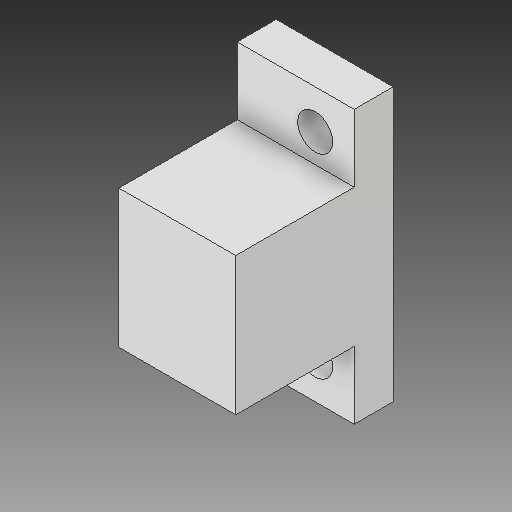
# Autodesk Inventor part: RailMount
Saved by Autodesk Inventor 2019.3 (Build 233278000, 278)
## iProperties
Created: 2019-06-25
Part Number: RailMount
Material: PC/ABS Plastic
Document SubType Name: Modeling
Designer: mark
Density: 0.357273 g/cm^3
Appearance: Smooth - White
Author: mark
Autodesk Inventor part; units mm, degrees
ref_plane "YZ Plane" through (0, 0, 0) normal (1, 0, 0) x (0, 1, 0)
ref_plane "XZ Plane" through (0, 0, 0) normal (0, 1, 0) x (-1, 0, 0)
ref_plane "XY Plane" through (0, 0, 0) normal (0, 0, 1) x (1, 0, 0)
sketch "Sketch1" plane through (0, 0, 0) normal (0, 0, 1) x (1, 0, 0)
  circle A0 centre (-50, 5.188) radius 4.5 projected
  circle A1 centre (-50, -44.812) radius 4.5 projected
  circle A2 centre (50, 5.188) radius 4.5 projected
  circle A3 centre (50, -44.812) radius 4.5 projected
  line L0 (30, 15.188) -> (60, 15.188)
  line L1 (60, 15.188) -> (60, -54.812)
  line L2 (60, -54.812) -> (30, -54.812)
  line L3 (30, -54.812) -> (30, 15.188)
  circle A4 centre (50, 5.188) radius 4
  circle A5 centre (50, -44.812) radius 4
  point P0 (0, 0)
  dimension "d1" = 30
  dimension "d2" = 60
  dimension "d28" = 10
  dimension "d29" = 10
  constraints: 8 end point, 2 centre point, 2 coincident, 2 horizontal, 2 vertical
  measures "d1" distance between parallel lines of L1 L3
  measures "d2" distance from line of point (0, 0) L1
  measures "d28" distance from line of L0 A2.centre
  measures "d29" distance from line of L2 A3.centre
extrude "Extrusion1" add sketch "Sketch1" along normal blind 10 contours L0 L1 L2 L3
sketch "Sketch2" plane through (0, 0, 10) normal (0, 0, 1) x (1, 0, 0)
  line L0 (60, -2.112) -> (55, -2.112)
  line L1 (55, -2.112) -> (55, -37.512)
  line L2 (55, -37.512) -> (60, -37.512)
  line L3 (60, -37.512) -> (60, -2.112)
  line L4 (60, 15.188) -> (30, 15.188) projected
  line L5 (30, -54.812) -> (60, -54.812) projected
  line L6 (60, -54.812) -> (60, 15.188) projected
  point P0 (0, 0)
  dimension "d7" = 5
  dimension "d26" = 35.4
  dimension "d27" = 17.3
  constraints: 8 end point, 1 collinear
  measures "d7" distance between parallel lines of L1 L3
  measures "d26" distance between parallel lines of L2 L0
  measures "d27" distance between parallel lines of L0 L4
extrude "Extrusion2" add sketch "Sketch2" along normal blind 30.4
sketch "Sketch3" plane through (55, -37.512, 10) normal (-1, 0, 0) x (0, 0, 1)
  line L0 (30.4, 35.4) -> (0, 35.4)
  line L1 (0, 35.4) -> (0, 30.4)
  line L2 (0, 30.4) -> (30.4, 30.4)
  line L3 (30.4, 30.4) -> (30.4, 35.4)
  line L4 (30.4, 5) -> (25.4, 5)
  line L5 (25.4, 5) -> (25.4, 30.4)
  line L6 (25.4, 30.4) -> (30.4, 30.4)
  line L7 (30.4, 30.4) -> (30.4, 5)
  line L8 (30.4, 0) -> (0, 0)
  line L9 (0, 0) -> (0, 5)
  line L10 (0, 5) -> (30.4, 5)
  line L11 (30.4, 5) -> (30.4, 0)
  line L12 (0, 52.7) -> (0, -17.3) projected
  line L13 (30.4, 35.4) -> (30.4, 0) projected
  line L14 (0, 35.4) -> (30.4, 35.4) projected
  dimension "d21" = 25.4
  dimension "d22" = 25.4
  dimension "d23" = 5
  dimension "d24" = 5
  constraints: 24 end point, 8 collinear
  measures "d21" distance between parallel lines of L10 L2
  measures "d22" distance between parallel lines of L12 L5
  measures "d23" distance between parallel lines of L2 L0
  measures "d24" distance between parallel lines of L8 L4
extrude "Extrusion3" add sketch "Sketch3" along normal up to surface (25 mm away) contours L3 L2 L1 L0 | L7 L4 L5 L2 | L11 L8 L9 L10 L4
body "Solid1"
